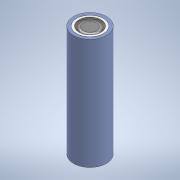
# Autodesk Inventor part: baterka
Saved by Autodesk Inventor 2022 (Build 260153000, 153)
## iProperties
Created: 2022-11-28
Part Number: baterka
Material: Generic
Document SubType Name: Modeling
Designer: matys
Density: 1 g/cm^3
Appearance: Default
Author: matys
Autodesk Inventor part; units mm, degrees
ref_plane "YZ Plane" through (0, 0, 0) normal (1, 0, 0) x (0, 1, 0)
ref_plane "XZ Plane" through (0, 0, 0) normal (0, 1, 0) x (-1, 0, 0)
ref_plane "XY Plane" through (0, 0, 0) normal (0, 0, 1) x (1, 0, 0)
sketch "Sketch1" plane through (0, 0, 0) normal (0, 1, 0) x (-1, 0, 0)
  circle A0 centre (0, 0) radius 10.5
  dimension "d0" = 21
  constraints: 1 centre point, 1 coincident
  measures "d0" diameter of A0
extrude "Extrusion1" add sketch "Sketch1" along normal blind 70.8
sketch "Sketch2" plane through (0, 70.8, 0) normal (0, 1, 0) x (1, 0, 0)
  circle A0 centre (0, 0) radius 10.5 projected
  line L0 (-10.5, 0) -> (-7, 0)
  circle A1 centre (0, 0) radius 7
  dimension "d3" = 3.5
  constraints: 2 end point, 2 horizontal alignment, 1 coincident, 1 horizontal, 3 other
  measures "d3" distance of L0.start L0.end
extrude "Extrusion2" cut sketch "Sketch2" against normal blind 2 contours A1
sketch "Sketch3" plane through (0, 68.8, 0) normal (0, 1, 0) x (1, 0, 0)
  circle A0 centre (0, 0) radius 10.5 projected
  line L0 (-10.5, 0) -> (-8.5, 0)
  circle A1 centre (0, 0) radius 8.5
  dimension "d6" = 2
  constraints: 2 end point, 2 horizontal alignment, 1 coincident, 1 horizontal, 3 other
  measures "d6" distance of L0.start L0.end
extrude "Extrusion3" cut sketch "Sketch3" along normal blind 1.75 contours A1
sketch "Sketch4" plane through (0, 68.8, 0) normal (0, 1, 0) x (1, 0, 0)
  circle A0 centre (0, 0) radius 5.75
  dimension "d9" = 11.5
  constraints: 1 centre point, 1 coincident
  measures "d9" diameter of A0
extrude "Extrusion4" add sketch "Sketch4" along normal blind 1.5
fillet "Fillet1" radius 1.5 1 edges at (-5.75, 70.3, 0)
sketch "Sketch5" plane through (0, 70.8, 0) normal (0, 1, 0) x (1, 0, 0)
  circle A0 centre (0, 0) radius 7
  circle A1 centre (0, 0) radius 7 projected
  line L0 (0, 7) -> (0, 8.5)
  circle A2 centre (0, 0) radius 8.5 projected
  circle A3 centre (0, 0) radius 4.25 projected
  circle A4 centre (0, 0) radius 8.5
  constraints: 2 centre point, 2 coincident, 2 end point, 2 vertical alignment, 1 vertical, 3 other
extrude "Extrusion5" cut sketch "Sketch5" against normal blind 0.05 contours A2
sketch "Sketch6" plane through (0, 0, 0) normal (0, -1, 0) x (1, 0, 0)
  circle A0 centre (0, 0) radius 10.5 projected
  line L0 (0, 10.5) -> (0, 8.5)
  circle A1 centre (0, 0) radius 8.5 projected
  circle A2 centre (0, 0) radius 8.5
  circle A3 centre (0, 0) radius 10.5
  constraints: 4 vertical alignment, 2 coincident, 2 end point, 1 vertical, 6 other
extrude "Extrusion6" cut sketch "Sketch6" against normal blind 0.05 contours A1
body "Solid1"
